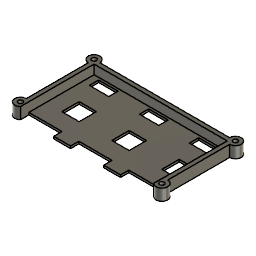
sensor_holder (Autodesk Fusion 360 design; units mm, degrees)
part number: 2026-04-05-13-06-35-929
Autodesk Fusion 360 part; units mm, degrees
sketch "Sketch1" plane through (0, 0, 0) normal (0, 0, 1) x (1, 0, 0)
  line L0 (0, 0) -> (18, 0)
  line L1 (18, 0) -> (18, 32)
  line L2 (18, 32) -> (0, 32)
  line L3 (0, 32) -> (0, 0)
  line L4 (1.8, 1.8) -> (16.2, 1.8)
  line L5 (16.2, 1.8) -> (16.2, 30.2)
  line L6 (16.2, 30.2) -> (1.8, 30.2)
  line L7 (1.8, 30.2) -> (1.8, 1.8)
  line L8 (1.8, 1.8) -> (1.8, 0)
  line L9 (16.2, 1.8) -> (16.2, 0)
  line L10 (1.8, 0) -> (1.8, -1.8)
  line L11 (16.2, 0) -> (16.2, -1.8)
  line L12 (16.2, 1.8) -> (18, 1.8)
  dimension "d1" = 18
  dimension "d2" = 32
  dimension "d3" = 28.4
  dimension "d4" = 14.4
  dimension "d5" = 1.8
  dimension "d6" = 1.8
  constraint horizontal L0
  constraint vertical L1
  constraint horizontal L2
  constraint vertical L3
  constraint coincident L0.start L3.end
  constraint horizontal L4
  constraint vertical L5
  constraint horizontal L6
  constraint vertical L7
  constraint coincident L0 L8.end
  constraint perpendicular L0 L8
  constraint coincident L0 L9.end
  constraint perpendicular L0 L9
  constraint perpendicular L0 L10
  constraint perpendicular L0 L11
  constraint coincident L1 L12.end
  constraint perpendicular L1 L12
  measures "d1" distance of L0.start L0.end
  measures "d2" distance of L0.start L2.end
  measures "d3" distance of L4.start L6.end
  measures "d4" distance of L4.start L4.end
  measures "d5" distance of L2 L6
  measures "d6" distance of L1 L5
extrude "Extrude1" add sketch "Sketch1" along normal blind 1 contours L4 L5 L6 L7 makes body 1
extrude "Extrude3" add sketch "Sketch1" along normal blind 5 separate body contours L0 L1 L2 L3 L5 L6 L7 L8 L12 | L0 L1 L9 L12 makes body 2
sketch "Sketch3" plane through (0, 30.2, 0) normal (0, -1, 0) x (1, 0, 0)
  line L0 (1.8, 0) -> (16.2, 0)
  line L1 (16.2, 0) -> (16.2, 5)
  line L2 (16.2, 5) -> (1.8, 5)
  line L3 (1.8, 5) -> (1.8, 0)
  line L4 (3.3, 1) -> (14.7, 1)
  line L5 (14.7, 1) -> (14.7, 4)
  line L6 (14.7, 4) -> (3.3, 4)
  line L7 (3.3, 4) -> (3.3, 1)
  dimension "d13" = 3
  dimension "d14" = 1.5
  dimension "d15" = 1.5
  constraint horizontal L4
  constraint vertical L5
  constraint horizontal L6
  constraint vertical L7
  measures "d13" distance of L4.start L6.end
  measures "d14" distance of L1 L5
  measures "d15" distance of L3 L7
sketch "Sketch4" plane through (0, 0, 1) normal (0, 0, 1) x (-1, 0, 0)
  line L0 (-1.8, -30.2) -> (-1.8, -1.8)
  line L1 (-1.8, -1.8) -> (-16.2, -1.8)
  line L2 (-16.2, -1.8) -> (-16.2, -30.2)
  line L3 (-16.2, -30.2) -> (-1.8, -30.2)
  line L4 (-13.5403, -1.8) -> (-13.5403, -9.3)
  line L5 (-16.2, -9.3) -> (-8.7, -9.3)
  line L6 (-8.7, -9.3) -> (-8.7, -16.8)
  line L7 (-8.7, -16.8) -> (-16.2, -16.8)
  line L8 (-16.2, -16.8) -> (-16.2, -9.3)
  dimension "d18" = 7.5
  dimension "d19" = 7.5
  dimension "d20" = 7.5
  constraint coincident L1 L4.start
  constraint perpendicular L1 L4
  constraint coincident L2 L5.start
  constraint perpendicular L2 L5
  constraint perpendicular L5 L6
  constraint coincident L2 L7.end
  constraint perpendicular L2 L7
  constraint coincident L4.end L5
  measures "d18" distance of L4.start L4.end
  measures "d19" distance of L5.start L5.end
  measures "d20" distance of L5.end L6.end
extrude "Extrude5" cut sketch "Sketch4" against normal blind 1 contours L2 L5 L6 L7 L8 bodies 1
sketch "Sketch5" plane through (0, 0, 1) normal (0, 0, 1) x (-1, 0, 0)
  line L0 (-8.7, -16.8) -> (-16.2, -16.8)
  line L1 (-16.2, -16.8) -> (-16.2, -30.2)
  line L2 (-16.2, -30.2) -> (-1.8, -30.2)
  line L3 (-1.8, -30.2) -> (-1.8, -1.8)
  line L4 (-1.8, -1.8) -> (-16.2, -1.8)
  line L5 (-16.2, -1.8) -> (-16.2, -9.3)
  line L6 (-16.2, -9.3) -> (-8.7, -9.3)
  line L7 (-8.7, -9.3) -> (-8.7, -16.8)
  line L8 (-9, -30.2) -> (-9, -25.2) construction
  line L9 (-1.8, -25.2) -> (-4.8, -25.2) construction
  line L10 (-16.2, -25.2) -> (-13.2, -25.2) construction
  line L11 (-8.3545, -30.2) -> (-8.3545, -29.2)
  line L12 (-13.2, -25.2) -> (-4.8, -25.2)
  line L13 (-4.8, -25.2) -> (-4.8, -29.2)
  line L14 (-4.8, -29.2) -> (-13.2, -29.2)
  line L15 (-13.2, -29.2) -> (-13.2, -25.2)
  dimension "d24" = 3
  dimension "d25" = 3
  dimension "d26" = 1
  dimension "d27" = 5
  dimension "d28" = 4
  constraint midpoint L2 L8.start
  constraint perpendicular L2 L8
  constraint coincident L3 L9.start
  constraint perpendicular L3 L9
  constraint coincident L1 L10.start
  constraint perpendicular L1 L10
  constraint coincident L2 L11.start
  constraint perpendicular L2 L11
  constraint horizontal L12
  constraint midpoint L12 L8.end
  constraint coincident L12.start L10
  constraint coincident L9.end L12.end
  constraint perpendicular L12 L13
  constraint perpendicular L13 L14
  constraint perpendicular L14 L15
  measures "d24" distance of L9.start L9.end
  measures "d25" distance of L10.start L10.end
  measures "d26" distance of L11.start L11.end
  measures "d27" distance of L8.start L8.end
  measures "d28" distance of L9.end L13.end
sketch "Sketch7" plane through (0, 0, 5) normal (0, 0, 1) x (-1, 0, 0)
  line L0 (-16.2, -30.2) -> (-16.2, 0)
  line L1 (-16.2, 0) -> (-18, 0)
  line L2 (-18, 0) -> (-18, -32)
  line L3 (-18, -32) -> (0, -32)
  line L4 (0, -32) -> (0, 0)
  line L5 (0, 0) -> (-1.8, 0)
  line L6 (-1.8, 0) -> (-1.8, -30.2)
  line L7 (-1.8, -30.2) -> (-16.2, -30.2)
  line L8 (-16.2, -30.2) -> (-18, -30.2)
  line L9 (-16.2, 0) -> (-18, 0)
  constraint coincident L0.start L7.end
  constraint coincident L2 L8.end
  constraint perpendicular L2 L8
  constraint coincident L0.end L1.start
  constraint coincident L1.end L2.start
extrude "Extrude9" cut sketch "Sketch7" against normal blind 4 contours L0 L1 L2 L8 L9 bodies 2
combine "Combine2" operation add target body 2 tool bodies 1
extrude "Extrude6" cut sketch "Sketch5" against normal blind 1 contours L12 L13 L14 L15 bodies 2
sketch "Sketch9" plane through (0, 0, 1) normal (0, 0, 1) x (-1, 0, 0)
  line L0 (-4.8, -25.2) -> (-4.8, -29.2)
  line L1 (-4.8, -29.2) -> (-13.2, -29.2)
  line L2 (-13.2, -29.2) -> (-13.2, -25.2)
  line L3 (-13.2, -25.2) -> (-4.8, -25.2)
  line L4 (-16.2, -1.8) -> (-16.2, 0)
  line L5 (-16.2, 0) -> (-18, 0)
  line L6 (-18, 0) -> (-18, -30.2)
  line L7 (-18, -30.2) -> (-1.8, -30.2)
  line L8 (-1.8, -30.2) -> (-1.8, -1.8)
  line L9 (-1.8, -1.8) -> (-16.2, -1.8)
  line L10 (-16.2, -9.3) -> (-8.7, -9.3)
  line L11 (-8.7, -9.3) -> (-8.7, -16.8)
  line L12 (-8.7, -16.8) -> (-16.2, -16.8)
  line L13 (-16.2, -16.8) -> (-16.2, -9.3)
  line L14 (-9, -34.6502) -> (-30.75, -34.6502)
  line L15 (-30.75, -34.6502) -> (-52.5, -34.6502)
  line L16 (-52.5, -34.6502) -> (-59.7, -34.6502)
  line L17 (-59.7, -34.6502) -> (-61.5, -34.6502)
  line L18 (-18, -32) -> (-61.5, -32)
  line L19 (-61.5, -32) -> (-61.5, 0)
  line L20 (-61.5, 0) -> (-18, 0)
  line L21 (-18, 0) -> (-18, -32)
  line L22 (-9, -30.2) -> (-9, -25.2)
  line L23 (-18, -30.2) -> (-59.7, -30.2)
  line L24 (-59.7, -30.2) -> (-59.7, -1.8)
  line L25 (-59.7, -1.8) -> (-18, -1.8)
  line L26 (-18, -1.8) -> (-18, -30.2)
  line L27 (-59.7, -1.8) -> (-61.5, -1.8)
  line L28 (-41.625, -34.6502) -> (-41.625, -24)
  point P0 (-18, -32)
  dimension "d42" = 21.75
  dimension "d43" = 21.75
  dimension "d44" = 7.2
  dimension "d45" = 1.8
  dimension "d46" = 1.8
  dimension "d47" = 1.8
  constraint perpendicular L6 L14
  constraint parallel L14 L15
  constraint parallel L15 L16
  constraint parallel L16 L17
  constraint horizontal L18
  constraint vertical L19
  constraint horizontal L20
  constraint vertical L21
  constraint coincident L17.end L19
  constraint coincident L21 P0
  constraint coincident L5.end L20
  constraint coincident L14.start L22
  constraint coincident L18 P0
  constraint horizontal L23
  constraint vertical L24
  constraint horizontal L25
  constraint vertical L26
  constraint coincident L6.end L7.start
  constraint coincident L19 L27.end
  constraint perpendicular L19 L27
  constraint midpoint L15 L28.start
  constraint perpendicular L23 L28
  measures "d42" distance of L14.start L14.end
  measures "d43" distance of L14.end L15.end
  measures "d44" distance of L15.end L16.end
  measures "d45" distance of L16.end L17.end
  measures "d46" distance of L20 L25
  measures "d47" distance of L19 L24
extrude "Extrude12" add sketch "Sketch9" against normal blind 1 contours L6 L21 L23 L24 L25 L26 bodies 2
extrude "Extrude13" add sketch "Sketch9" along normal blind 4 contours L18 L21 L23 L28 | L18 L19 L23 L24 L27 L28 bodies 2
extrude "Extrude14" add sketch "Sketch9" along normal blind 1 contours L18 L21 L23 L28 | L18 L19 L23 L24 L27 L28 bodies 2
sketch "Sketch10" plane through (0, 0, 1) normal (0, 0, -1) x (1, 0, 0)
  line L0 (59.7, -30.2) -> (18, -30.2)
  line L1 (18, -30.2) -> (18, -32)
  line L2 (18, -32) -> (61.5, -32)
  line L3 (61.5, -32) -> (61.5, -1.8)
  line L4 (61.5, -1.8) -> (59.7, -1.8)
  line L5 (59.7, -1.8) -> (59.7, -30.2)
extrude "Extrude15" add 1 faces at (46.4, 31.4, 1) along direction (0, 0, -1) blind 1 on bodies 2 bodies 2
sketch "Sketch11" plane through (0, 0, 1) normal (0, 0, 1) x (-1, 0, 0)
  line L0 (-4.8, -25.2) -> (-4.8, -29.2)
  line L1 (-4.8, -29.2) -> (-13.2, -29.2)
  line L2 (-13.2, -29.2) -> (-13.2, -25.2)
  line L3 (-13.2, -25.2) -> (-4.8, -25.2)
  line L4 (-16.2, -1.8) -> (-16.2, 0)
  line L5 (-16.2, 0) -> (-18, 0)
  line L6 (-18, 0) -> (-18, -1.8)
  line L7 (-18, -1.8) -> (-59.7, -1.8)
  line L8 (-59.7, -1.8) -> (-59.7, -30.2)
  line L9 (-59.7, -30.2) -> (-1.8, -30.2)
  line L10 (-1.8, -30.2) -> (-1.8, -1.8)
  line L11 (-1.8, -1.8) -> (-16.2, -1.8)
  line L12 (-16.2, -9.3) -> (-8.7, -9.3)
  line L13 (-8.7, -9.3) -> (-8.7, -16.8)
  line L14 (-8.7, -16.8) -> (-16.2, -16.8)
  line L15 (-16.2, -16.8) -> (-16.2, -9.3)
  line L16 (-9, -34.6502) -> (-30.75, -34.6502)
  line L17 (-30.75, -34.6502) -> (-52.5, -34.6502)
  line L18 (-52.5, -34.6502) -> (-59.7, -34.6502)
  line L19 (-59.7, -34.6502) -> (-61.5, -34.6502)
  line L20 (-9, -30.2) -> (-9, -25.2)
  line L21 (-19.875, -34.6502) -> (-19.875, -25)
  line L22 (-41.625, -34.6502) -> (-41.625, -25)
  line L23 (-26.55, -25.2) -> (-34.95, -25.2)
  line L24 (-34.95, -29.2) -> (-26.55, -29.2)
  line L25 (-34.95, -25.2) -> (-34.95, -29.2)
  line L26 (-26.55, -29.2) -> (-26.55, -25.2)
  line L27 (-56.7, -25.2) -> (-48.3, -25.2)
  line L28 (-56.7, -29.2) -> (-56.7, -25.2)
  line L29 (-48.3, -29.2) -> (-56.7, -29.2)
  line L30 (-48.3, -25.2) -> (-48.3, -29.2)
  line L31 (-16.2, -1.8) -> (-18, -1.8)
  line L32 (-12.45, -25.1815) -> (-12.45, -9.3) construction
  line L33 (-34.2, -25.2) -> (-34.2, -21.3798)
  line L34 (-12.45, -25.1815) -> (-34.2, -25.2) construction
  line L35 (-23.325, -25.1907) -> (-23.325, -13.8088) construction
  line L36 (-34.2, -25.2) -> (-55.95, -25.2) construction
  line L37 (-45.075, -25.2) -> (-45.075, -12.6632) construction
  line L38 (-37.95, -16.8) -> (-30.45, -16.8)
  line L39 (-30.45, -16.8) -> (-30.45, -9.3)
  line L40 (-30.45, -9.3) -> (-37.95, -9.3)
  line L41 (-37.95, -9.3) -> (-37.95, -16.8)
  line L42 (-52.2, -16.8) -> (-59.7, -16.8)
  line L43 (-52.2, -9.3) -> (-52.2, -16.8)
  line L44 (-59.7, -9.3) -> (-52.2, -9.3)
  line L45 (-59.7, -16.8) -> (-59.7, -9.3)
  dimension "d64" = 0.75
  dimension "d65" = 21.75
  constraint midpoint L16 L21.start
  constraint perpendicular L9 L21
  constraint midpoint L17 L22.start
  constraint perpendicular L9 L22
  constraint symmetric L0.start L21 L23.end
  constraint symmetric L0.end L21 L24.start
  constraint symmetric L1.end L21 L24.end
  constraint symmetric L2.end L21 L23.start
  constraint symmetric L22 L23.start L27.start
  constraint symmetric L22 L23.end L27.end
  constraint symmetric L22 L24.start L29.start
  constraint symmetric L22 L24.end L28.start
  constraint coincident L4.start L11.end
  constraint coincident L6.end L7.start
  constraint midpoint L12 L32.end
  constraint perpendicular L3 L32
  constraint coincident L23 L33.start
  constraint perpendicular L23 L33
  constraint midpoint L34 L35.start
  constraint perpendicular L30 L36
  constraint midpoint L36 L37.start
  constraint perpendicular L36 L37
  constraint symmetric L12.start L35 L39.end
  constraint symmetric L12.end L35 L40.end
  constraint symmetric L13.end L35 L38.start
  constraint symmetric L14.end L35 L38.end
  constraint symmetric L37 L38.start L42.start
  constraint symmetric L37 L38.end L42.end
  constraint symmetric L37 L39.end L44.start
  constraint symmetric L37 L40.end L43.start
  measures "d64" distance of L25 L33
  measures "d65" distance of L33.start L36.end
extrude "Extrude16" cut sketch "Sketch11" against normal blind 1 contours L23 L24 L25 L26 | L27 L28 L29 L30 bodies 2
extrude "Extrude17" cut sketch "Sketch11" against normal blind 1 contours L4 L5 L6 L31 bodies 2
extrude "Extrude19" cut sketch "Sketch11" against normal blind 1 contours L8 L42 L43 L44 L45 | L38 L39 L40 L41 bodies 2
sketch "Sketch12" plane through (0, 0, 5) normal (0, 0, 1) x (-1, 0, 0)
  line L0 (-1.8, -30.2) -> (-59.7, -30.2)
  line L1 (-59.7, -30.2) -> (-59.7, -1.8)
  line L2 (-59.7, -1.8) -> (-61.5, -1.8)
  line L3 (-61.5, -1.8) -> (-61.5, -32)
  line L4 (-61.5, -32) -> (0, -32)
  line L5 (0, -32) -> (0, 0)
  line L6 (0, 0) -> (-1.8, 0)
  line L7 (-1.8, 0) -> (-1.8, -30.2)
  line L8 (-59.7, -1.8) -> (-61.5, -1.8)
  line L9 (-61.5, -1.8) -> (-61.5, 0)
  line L10 (-61.5, 0) -> (-59.7, 0)
  line L11 (-59.7, 0) -> (-59.7, -1.8)
  dimension "d70" = 1.8
  dimension "d71" = 1.8
  constraint horizontal L8
  constraint vertical L9
  constraint horizontal L10
  constraint vertical L11
  constraint coincident L1.end L2.start
  measures "d70" distance of L1.end L2.end
  measures "d71" distance of L1.end L10.end
extrude "Extrude20" add sketch "Sketch12" against normal blind 5 contours L2 L8 L9 L10 L11 bodies 2
sketch "Sketch13" plane through (0, 0, 5) normal (0, 0, 1) x (-1, 0, 0)
  line L0 (-1.8, -30.2) -> (-59.7, -30.2)
  line L1 (-59.7, -30.2) -> (-59.7, 0)
  line L2 (-59.7, 0) -> (-61.5, 0)
  line L3 (-61.5, 0) -> (-61.5, -32)
  line L4 (-61.5, -32) -> (0, -32)
  line L5 (0, -32) -> (0, 0)
  line L6 (0, 0) -> (-1.8, 0)
  line L7 (-1.8, 0) -> (-1.8, -30.2)
  line L8 (-1.8, -1.8) -> (-59.7, -1.8)
  circle A0 centre (0, 0) radius 2.5456
  circle A1 centre (0, -32) radius 2.5456
  circle A2 centre (-61.5, 0) radius 2.5456
  circle A3 centre (-61.5, -32) radius 2.5456
  circle A4 centre (-61.5, 0) radius 1
  circle A5 centre (-61.5, -32) radius 1
  circle A6 centre (0, 0) radius 1
  circle A7 centre (0, -32) radius 1
  line L9 (-1.8, -1.8) -> (-1.8, 1.8)
  line L10 (-59.6731, -1.7885) -> (-59.6731, 1.7727)
  dimension "d74" = 2
  dimension "d75" = 2
  dimension "d76" = 2
  dimension "d77" = 2
  constraint coincident L5.end L6.start
  constraint coincident L8.start A0
  constraint coincident L4.end L5.start
  constraint coincident L0.start A1
  constraint coincident L2.end L3.start
  constraint coincident L8.end A2
  constraint coincident L3.end L4.start
  constraint coincident L0.end A3
  constraint concentric A2 A4
  constraint concentric A3 A5
  constraint concentric A0 A6
  constraint coincident L8.start L9.start
  constraint coincident A0 L9.end
  constraint perpendicular L8 L9
  constraint coincident A2 L10.end
  constraint perpendicular L8 L10
  measures "d74" diameter of A4
  measures "d75" diameter of A5
  measures "d76" diameter of A6
  measures "d77" diameter of A7
extrude "Extrude21" add sketch "Sketch13" against normal blind 5 contours L4 L5 A1 A7 | L1 L2 L3 A2 A4 L10 | L3 L4 A3 A5 | L5 L6 A0 A6 L9 picked at (2.0172, -32.1761) picked at (-60.086, -33.4496) bodies 2
extrude "Extrude22" cut sketch "Sketch13" against normal blind 5 contours L4 L5 A7 | L3 L4 A5 | L5 L6 A6 | L2 L3 A4 picked at (-0.6633, -31.9526) picked at (-60.8502, -31.8587) picked at (-0.0474, -0.6633) picked at (-60.9677, -0.3985) bodies 2
sketch "Sketch14" plane through (0, 0, 1) normal (0, 0, 1) x (-1, 0, 0)
  line L0 (-52.2, -16.8) -> (-59.7, -16.8)
  line L1 (-59.7, -16.8) -> (-59.7, -30.2)
  line L2 (-59.7, -30.2) -> (-1.8, -30.2)
  line L3 (-1.8, -30.2) -> (-1.8, -1.8)
  line L4 (-1.8, -1.8) -> (-59.7, -1.8)
  line L5 (-59.7, -1.8) -> (-59.7, -9.3)
  line L6 (-59.7, -9.3) -> (-52.2, -9.3)
  line L7 (-52.2, -9.3) -> (-52.2, -16.8)
  line L8 (-30.45, -16.8) -> (-37.95, -16.8)
  line L9 (-37.95, -16.8) -> (-37.95, -9.3)
  line L10 (-37.95, -9.3) -> (-30.45, -9.3)
  line L11 (-30.45, -9.3) -> (-30.45, -16.8)
  line L12 (-34.95, -25.2) -> (-26.55, -25.2)
  line L13 (-26.55, -25.2) -> (-26.55, -29.2)
  line L14 (-26.55, -29.2) -> (-34.95, -29.2)
  line L15 (-34.95, -29.2) -> (-34.95, -25.2)
  line L16 (-56.7, -29.2) -> (-56.7, -25.2)
  line L17 (-56.7, -25.2) -> (-48.3, -25.2)
  line L18 (-48.3, -25.2) -> (-48.3, -29.2)
  line L19 (-48.3, -29.2) -> (-56.7, -29.2)
  line L20 (-4.8, -25.2) -> (-4.8, -29.2)
  line L21 (-4.8, -29.2) -> (-13.2, -29.2)
  line L22 (-13.2, -29.2) -> (-13.2, -25.2)
  line L23 (-13.2, -25.2) -> (-4.8, -25.2)
  line L24 (-16.2, -9.3) -> (-8.7, -9.3)
  line L25 (-8.7, -9.3) -> (-8.7, -16.8)
  line L26 (-8.7, -16.8) -> (-16.2, -16.8)
  line L27 (-16.2, -16.8) -> (-16.2, -9.3)
  line L28 (-13.2, -27.2) -> (-16.2, -27.2)
  line L29 (-16.2, -27.2) -> (-16.2, -1.8)
  line L30 (-16.2, -1.8) -> (-16.2, 1.8)
  line L31 (-26.55, -27.2) -> (-23.55, -27.2)
  line L32 (-16.2, 1.8) -> (-23.55, 1.8)
  line L33 (-23.55, 1.8) -> (-23.55, -1.8)
  line L34 (-30.75, -29.2) -> (-30.75, -25.2)
  line L35 (-16.2, -1.8) -> (-23.55, -1.8)
  line L36 (-37.95, 1.8) -> (-37.95, -1.8)
  line L37 (-45.3, -1.8) -> (-37.95, -1.8)
  line L38 (-45.3, 1.8) -> (-37.95, 1.8)
  line L39 (-45.3, -1.8) -> (-45.3, 1.8)
  dimension "d82" = 3
  dimension "d83" = 3.6
  dimension "d84" = 3
  dimension "d85" = 7.35
  constraint midpoint L22 L28.start
  constraint perpendicular L22 L28
  constraint coincident L4 L29.end
  constraint perpendicular L4 L29
  constraint perpendicular L4 L30
  constraint midpoint L13 L31.start
  constraint perpendicular L13 L31
  constraint perpendicular L30 L32
  constraint coincident L4 L33.end
  constraint perpendicular L4 L33
  constraint midpoint L14 L34.start
  constraint midpoint L12 L34.end
  constraint symmetric L29.end L34 L37.start
  constraint symmetric L30.end L34 L38.start
  constraint symmetric L32.end L34 L36.start
  constraint symmetric L33.end L34 L36.end
  measures "d82" distance of L28.start L28.end
  measures "d83" distance of L29.end L30.end
  measures "d84" distance of L31.start L31.end
  measures "d85" distance of L30.end L32.end
extrude "Extrude23" add sketch "Sketch14" against normal blind 1 contours L4 L36 L37 L38 L39 | L4 L30 L32 L33 L35 bodies 2
sketch "Sketch15" plane through (0, 0, 0) normal (0, 0, -1) x (1, 0, 0)
  line L0 (26.55, -25.2) -> (34.95, -25.2)
  line L1 (34.95, -25.2) -> (34.95, -29.2)
  line L2 (34.95, -29.2) -> (26.55, -29.2)
  line L3 (26.55, -29.2) -> (26.55, -25.2)
  line L4 (56.7, -25.2) -> (56.7, -29.2)
  line L5 (56.7, -29.2) -> (48.3, -29.2)
  line L6 (48.3, -29.2) -> (48.3, -25.2)
  line L7 (48.3, -25.2) -> (56.7, -25.2)
  line L8 (4.8, -29.2) -> (4.8, -25.2)
  line L9 (4.8, -25.2) -> (13.2, -25.2)
  line L10 (13.2, -25.2) -> (13.2, -29.2)
  line L11 (13.2, -29.2) -> (4.8, -29.2)
  line L12 (16.2, -9.3) -> (16.2, -16.8)
  line L13 (16.2, -16.8) -> (8.7, -16.8)
  line L14 (8.7, -16.8) -> (8.7, -9.3)
  line L15 (8.7, -9.3) -> (16.2, -9.3)
  line L16 (1.8, -1.8) -> (1.8, 1.8)
  arc A0 (1.8, 1.8) -> (0, -2.5456) centre (0, 0) ccw
  line L17 (0, -2.5456) -> (0, -29.4544)
  arc A1 (0, -29.4544) -> (2.5456, -32) centre (0, -32) ccw
  line L18 (2.5456, -32) -> (58.9544, -32)
  arc A2 (58.9544, -32) -> (61.5, -29.4544) centre (61.5, -32) ccw
  line L19 (61.5, -29.4544) -> (61.5, -2.5456)
  arc A3 (61.5, -2.5456) -> (59.6731, 1.7727) centre (61.5, 0) ccw
  line L20 (59.6731, 1.7727) -> (59.6731, -1.7727)
  arc A4 (59.6731, -1.7727) -> (59.7, -1.8) centre (61.5, 0) ccw
  line L21 (59.7, -1.8) -> (45.3, -1.8)
  line L22 (45.3, -1.8) -> (45.3, 1.8)
  line L23 (45.3, 1.8) -> (37.95, 1.8)
  line L24 (37.95, 1.8) -> (37.95, -1.8)
  line L25 (37.95, -1.8) -> (23.55, -1.8)
  line L26 (23.55, -1.8) -> (23.55, 1.8)
  line L27 (23.55, 1.8) -> (16.2, 1.8)
  line L28 (16.2, 1.8) -> (16.2, -1.8)
  line L29 (16.2, -1.8) -> (1.8, -1.8)
  line L30 (52.2, -16.8) -> (52.2, -9.3)
  line L31 (52.2, -9.3) -> (59.7, -9.3)
  line L32 (59.7, -9.3) -> (59.7, -16.8)
  line L33 (59.7, -16.8) -> (52.2, -16.8)
  line L34 (37.95, -16.8) -> (30.45, -16.8)
  line L35 (30.45, -16.8) -> (30.45, -9.3)
  line L36 (30.45, -9.3) -> (37.95, -9.3)
  line L37 (37.95, -9.3) -> (37.95, -16.8)
  circle A5 centre (0, -32) radius 1
  circle A6 centre (61.5, 0) radius 1
  circle A7 centre (0, 0) radius 1
  circle A8 centre (61.5, -32) radius 1
  line L38 (30.75, -29.2) -> (30.75, -25.2) construction
  line L39 (34.95, -27.2) -> (26.55, -27.2) construction
  circle A9 centre (30.75, -27.2) radius 1
  dimension "d88" = 2
  constraint midpoint L2 L38.start
  constraint midpoint L0 L38.end
  constraint midpoint L1 L39.start
  constraint midpoint L3 L39.end
  constraint midpoint L38 A9.centre
  measures "d88" diameter of A9
sketch "Sketch16" plane through (0, 0, 1) normal (0, 0, 1) x (-1, 0, 0)
  line L0 (-52.2, -16.8) -> (-59.7, -16.8)
  line L1 (-59.7, -16.8) -> (-59.7, -30.2)
  line L2 (-59.7, -30.2) -> (-1.8, -30.2)
  line L3 (-1.8, -30.2) -> (-1.8, -1.8)
  line L4 (-1.8, -1.8) -> (-16.2, -1.8)
  line L5 (-16.2, -1.8) -> (-16.2, 1.8)
  line L6 (-16.2, 1.8) -> (-23.55, 1.8)
  line L7 (-23.55, 1.8) -> (-23.55, -1.8)
  line L8 (-23.55, -1.8) -> (-37.95, -1.8)
  line L9 (-37.95, -1.8) -> (-37.95, 1.8)
  line L10 (-37.95, 1.8) -> (-45.3, 1.8)
  line L11 (-45.3, 1.8) -> (-45.3, -1.8)
  line L12 (-45.3, -1.8) -> (-59.7, -1.8)
  line L13 (-59.7, -1.8) -> (-59.7, -9.3)
  line L14 (-59.7, -9.3) -> (-52.2, -9.3)
  line L15 (-52.2, -9.3) -> (-52.2, -16.8)
  line L16 (-30.45, -16.8) -> (-37.95, -16.8)
  line L17 (-37.95, -16.8) -> (-37.95, -9.3)
  line L18 (-37.95, -9.3) -> (-30.45, -9.3)
  line L19 (-30.45, -9.3) -> (-30.45, -16.8)
  line L20 (-34.95, -25.2) -> (-26.55, -25.2)
  line L21 (-26.55, -25.2) -> (-26.55, -29.2)
  line L22 (-26.55, -29.2) -> (-34.95, -29.2)
  line L23 (-34.95, -29.2) -> (-34.95, -25.2)
  line L24 (-56.7, -29.2) -> (-56.7, -25.2)
  line L25 (-56.7, -25.2) -> (-48.3, -25.2)
  line L26 (-48.3, -25.2) -> (-48.3, -29.2)
  line L27 (-48.3, -29.2) -> (-56.7, -29.2)
  line L28 (-4.8, -25.2) -> (-4.8, -29.2)
  line L29 (-4.8, -29.2) -> (-13.2, -29.2)
  line L30 (-13.2, -29.2) -> (-13.2, -25.2)
  line L31 (-13.2, -25.2) -> (-4.8, -25.2)
  line L32 (-16.2, -9.3) -> (-8.7, -9.3)
  line L33 (-8.7, -9.3) -> (-8.7, -16.8)
  line L34 (-8.7, -16.8) -> (-16.2, -16.8)
  line L35 (-16.2, -16.8) -> (-16.2, -9.3)
  line L36 (-34.2, -16.8) -> (-34.2, -9.3) construction
  line L37 (-30.45, -13.05) -> (-37.95, -13.05) construction
  circle A0 centre (-34.2, -13.05) radius 1
  dimension "d89" = 2
  constraint midpoint L16 L36.start
  constraint midpoint L18 L36.end
  constraint midpoint L19 L37.start
  constraint midpoint L17 L37.end
  constraint midpoint L36 A0.centre
  measures "d89" diameter of A0
